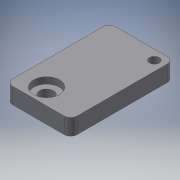
# Autodesk Inventor part: PinionHolderTest
Saved by Autodesk Inventor 2019 (Build 230136000, 136)
## iProperties
Created: 2019-08-06
Part Number: PinionHolderTest
Material: Generic
Document SubType Name: Modeling
Designer: aorfi
Density: 1 g/cm^3
Appearance: Default
Author: aorfi
Autodesk Inventor part; units mm, degrees
ref_plane "YZ Plane" through (0, 0, 0) normal (1, 0, 0) x (0, 1, 0)
ref_plane "XZ Plane" through (0, 0, 0) normal (0, 1, 0) x (-1, 0, 0)
ref_plane "XY Plane" through (0, 0, 0) normal (0, 0, 1) x (1, 0, 0)
sketch "Sketch1" plane through (0, 0, 0) normal (0, 1, 0) x (-1, 0, 0)
  line L0 (10, 17.5) -> (-10, 17.5)
  line L1 (-10, 17.5) -> (-10, -17.5)
  line L2 (-10, -17.5) -> (10, -17.5)
  line L3 (10, -17.5) -> (10, 17.5)
  line L4 (10, 17.5) -> (-10, -17.5) construction
  line L5 (-10, 17.5) -> (10, -17.5) construction
  point P0 (0, 0)
  dimension "d2" = 20
  dimension "d3" = 35
  constraints: 12 end point, 2 midpoint, 2 parallel, 1 horizontal, 1 perpendicular
  measures "d2" distance of L1.end L2.end
  measures "d3" distance of L0.end L1.end
extrude "Extrusion1" add sketch "Sketch1" along normal mid plane 5
sketch "Sketch3" plane through (0, 2.5, 0) normal (0, 1, 0) x (1, 0, 0)
  line L0 (-10, 17.5) -> (-10, -17.5) projected
  line L1 (10, -17.5) -> (10, 17.5) projected
  line L2 (-10, -17.5) -> (10, -17.5) projected
  line L3 (10, 17.5) -> (-10, 17.5) projected
  point P0 (0, 0)
  point P1 (-2.5, -9.5)
  point P2 (-10, 0)
  dimension "d26" = 12.5
  dimension "d28" = 8
  constraints: 1 midpoint
  measures "d26" distance from line of L1 point (-2.5, -9.5)
  measures "d28" distance from line of L2 point (-2.5, -9.5)
hole "Hole1" at (-2.5, 2.5, 9.5) direction (0, -1, 0) diameter 4.305 end through all clearance for "Flat Head Machine Screw (82)" size "#6" standard "Ansi Unified Screw Threads"
sketch "Sketch4" plane through (0, -2.5, 0) normal (0, -1, 0) x (1, 0, 0)
  circle A0 centre (-2.5, -6.977) radius 3.81
  circle A1 centre (-2.5, 9.5) radius 2.1525 projected
  point P0 (0, 0)
  dimension "d16" = 7.62
  dimension "d17" = 16.477
  constraints: 1 centre point, 1 vertical alignment
  measures "d16" diameter of A0
  measures "d17" distance of A0.centre A1.centre
extrude "Extrusion3" add sketch "Sketch4" along normal blind 5 contours A0
sketch "Sketch5" plane through (0, -2.5, 0) normal (0, -1, 0) x (1, 0, 0)
  circle A0 centre (7, -14.5) radius 1.5
  line L0 (-10, -17.5) -> (10, -17.5) projected
  line L1 (-10, 17.5) -> (-10, -17.5) projected
  line L2 (10, -17.5) -> (10, 17.5) projected
  circle A1 centre (-2.5, -6.977) radius 3.81 projected
  circle A2 centre (-2.5, 9.5) radius 2.1525 projected
  line L3 (10, 17.5) -> (-10, 17.5) projected
  line L4 (-10, 17.5) -> (-10, -17.5) projected
  line L5 (-10, -17.5) -> (10, -17.5) projected
  line L6 (10, -17.5) -> (10, 17.5) projected
  point P0 (0, 0)
  dimension "d20" = 3
  dimension "d33" = 7.523
  dimension "d34" = 9.5
  constraints: 1 centre point
  measures "d20" diameter of A0
  measures "d33" vertical distance of A1.centre A0.centre
  measures "d34" horizontal distance of A1.centre A0.centre
extrude "Extrusion4" cut sketch "Sketch5" against normal through all contours A0
sketch "Sketch6" plane through (0, 2.5, 0) normal (0, 1, 0) x (1, 0, 0)
  circle A0 centre (-2.5, -9.5) radius 2.1525 projected
  circle A1 centre (-2.5, -9.5) radius 4
  point P0 (0, 0)
  dimension "d30" = 8
  constraints: 1 centre point, 1 coincident
  measures "d30" diameter of A1
extrude "Extrusion5" cut sketch "Sketch6" against normal blind 2
sketch "Sketch7" plane through (0, -2.5, 0) normal (0, -1, 0) x (1, 0, 0)
  line L0 (10, 17.5) -> (10, -17.5) projected
  line L1 (10, 17.5) -> (-10, 17.5)
  line L2 (-10, 17.5) -> (-10, 14.5)
  line L3 (-10, 14.5) -> (10, 14.5)
  line L4 (10, 14.5) -> (10, 17.5)
  line L5 (-10, 17.5) -> (-10, -17.5) projected
  point P0 (0, 0)
  dimension "d35" = 3
  constraints: 8 end point, 2 parallel, 1 collinear, 1 horizontal, 1 perpendicular
  measures "d35" distance between parallel lines of L1 L3
extrude "Extrusion6" add sketch "Sketch7" along normal blind 2
fillet "Fillet1" radius 2 4 edges at (10, -1, 17.5) (-10, -1, 17.5) (10, 0, -17.5) (-10, 0, -17.5)
body "Solid1"
